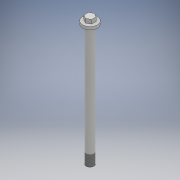
# Autodesk Inventor part: 前輪シャフト
Saved by Autodesk Inventor 2018 (Build 220112000, 112)
## iProperties
Created: 2017-09-10
Part Number: 前輪シャフト
Material: 一般
Document SubType Name: Modeling
Designer: mura5
Density: 1 g/cm^3
Appearance: 既定
Author: mura5
Autodesk Inventor part; units mm, degrees
ref_plane "YZ Plane" through (0, 0, 0) normal (1, 0, 0) x (0, 1, 0)
ref_plane "XZ Plane" through (0, 0, 0) normal (0, 1, 0) x (-1, 0, 0)
ref_plane "XY Plane" through (0, 0, 0) normal (0, 0, 1) x (1, 0, 0)
sketch "スケッチ1" plane through (0, 0, 0) normal (0, 0, 1) x (1, 0, 0)
  circle A0 centre (0, 0) radius 5.95
  dimension "d0" = 11.9
  constraints: 1 centre point, 1 coincident
  measures "d0" diameter of A0
extrude "押し出し1" add sketch "スケッチ1" along normal blind 188
thread "ねじ1" size "M12x1.75" class "6g" standard "ANSI Metric M Profile" length 17
sketch "スケッチ3" plane through (0, 0, 188) normal (0, 0, 1) x (1, 0, 0)
  circle A0 centre (0, 0) radius 11.3
  dimension "d5" = 22.6
  constraints: 1 centre point, 1 coincident
  measures "d5" diameter of A0
extrude "押し出し2" add sketch "スケッチ3" along normal blind 4.5
sketch "スケッチ4" plane through (0, 0, 192.5) normal (0, 0, 1) x (1, 0, 0)
  circle A0 centre (0, 0) radius 5.95 construction
  line L0 (5.95, -3.4352) -> (0, -6.8705)
  line L1 (0, -6.8705) -> (-5.95, -3.4352)
  line L2 (-5.95, -3.4352) -> (-5.95, 3.4352)
  line L3 (-5.95, 3.4352) -> (0, 6.8705)
  line L4 (0, 6.8705) -> (5.95, 3.4352)
  line L5 (5.95, 3.4352) -> (5.95, -3.4352)
  point P0 (5.95, 0)
  constraints: 12 end point, 1 horizontal alignment, 1 midpoint, 14 other
extrude "押し出し3" add sketch "スケッチ4" along normal blind 6.3
